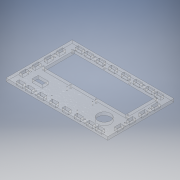
# Autodesk Inventor part: case_top
Saved by Autodesk Inventor 2019 (Build 230136000, 136)
## iProperties
Created: 2019-02-02
Part Number: case_top
Material: Acrylic, Clear
Document SubType Name: Modeling
Designer: suchanek
Density: 1.19 g/cm^3
Appearance: Transparent - Clear
Author: suchanek
Autodesk Inventor part; units mm, degrees
ref_plane "YZ Plane" through (0, 0, 0) normal (1, 0, 0) x (0, 1, 0)
ref_plane "XZ Plane" through (0, 0, 0) normal (0, 1, 0) x (-1, 0, 0)
ref_plane "XY Plane" through (0, 0, 0) normal (0, 0, 1) x (1, 0, 0)
sketch "Sketch1" plane through (0, 0, 0) normal (0, 1, 0) x (-1, 0, 0)
  line L0 (100, 65) -> (-100, 65)
  line L1 (-100, 65) -> (-100, -65)
  line L2 (-100, -65) -> (100, -65)
  line L3 (100, -65) -> (100, 65)
  line L4 (100, 65) -> (-100, -65) construction
  line L5 (-100, 65) -> (100, -65) construction
  line L6 (0, 0) -> (4.5236, 0)
  line L7 (0, 8) -> (0, -20)
  line L8 (0, 0) -> (5.2635, 0)
  line L9 (96, -42) -> (90, -42)
  line L10 (90, -42) -> (90, -30)
  line L11 (90, -30) -> (96, -30)
  line L12 (96, -30) -> (96, -42)
  line L13 (96, -18) -> (90, -18)
  line L14 (90, -18) -> (90, -6)
  line L15 (90, -6) -> (96, -6)
  line L16 (96, -6) -> (96, -18)
  line L17 (66, -55) -> (54, -55)
  line L18 (54, -55) -> (54, -61)
  line L19 (54, -61) -> (66, -61)
  line L20 (66, -61) -> (66, -55)
  line L21 (42, -55) -> (30, -55)
  line L22 (30, -55) -> (30, -61)
  line L23 (30, -61) -> (42, -61)
  line L24 (42, -61) -> (42, -55)
  line L25 (18, -55) -> (6, -55)
  line L26 (6, -55) -> (6, -61)
  line L27 (6, -61) -> (18, -61)
  line L28 (18, -61) -> (18, -55)
  line L29 (72, -61) -> (84, -61)
  line L30 (84, -61) -> (84, -55)
  line L31 (84, -55) -> (72, -55)
  line L32 (72, -55) -> (72, -61)
  line L33 (-96, -42) -> (-90, -42)
  line L34 (-90, -42) -> (-90, -30)
  line L35 (-90, -30) -> (-96, -30)
  line L36 (-96, -30) -> (-96, -42)
  line L37 (-96, -18) -> (-90, -18)
  line L38 (-90, -18) -> (-90, -6)
  line L39 (-90, -6) -> (-96, -6)
  line L40 (-96, -6) -> (-96, -18)
  line L41 (-66, -55) -> (-54, -55)
  line L42 (-54, -55) -> (-54, -61)
  line L43 (-54, -61) -> (-66, -61)
  line L44 (-66, -61) -> (-66, -55)
  line L45 (-42, -55) -> (-30, -55)
  line L46 (-30, -55) -> (-30, -61)
  line L47 (-30, -61) -> (-42, -61)
  line L48 (-42, -61) -> (-42, -55)
  line L49 (-18, -55) -> (-6, -55)
  line L50 (-6, -55) -> (-6, -61)
  line L51 (-6, -61) -> (-18, -61)
  line L52 (-18, -61) -> (-18, -55)
  line L53 (-72, -61) -> (-84, -61)
  line L54 (-84, -61) -> (-84, -55)
  line L55 (-84, -55) -> (-72, -55)
  line L56 (-72, -55) -> (-72, -61)
  line L57 (96, 42) -> (90, 42)
  line L58 (90, 42) -> (90, 30)
  line L59 (90, 30) -> (96, 30)
  line L60 (96, 30) -> (96, 42)
  line L61 (96, 18) -> (90, 18)
  line L62 (90, 18) -> (90, 6)
  line L63 (90, 6) -> (96, 6)
  line L64 (96, 6) -> (96, 18)
  line L65 (66, 55) -> (54, 55)
  line L66 (54, 55) -> (54, 61)
  line L67 (54, 61) -> (66, 61)
  line L68 (66, 61) -> (66, 55)
  line L69 (42, 55) -> (30, 55)
  line L70 (30, 55) -> (30, 61)
  line L71 (30, 61) -> (42, 61)
  line L72 (42, 61) -> (42, 55)
  line L73 (18, 55) -> (6, 55)
  line L74 (6, 55) -> (6, 61)
  line L75 (6, 61) -> (18, 61)
  line L76 (18, 61) -> (18, 55)
  line L77 (72, 61) -> (84, 61)
  line L78 (84, 61) -> (84, 55)
  line L79 (84, 55) -> (72, 55)
  line L80 (72, 55) -> (72, 61)
  line L81 (-90, 30) -> (-96, 30)
  line L82 (-96, 18) -> (-90, 18)
  line L83 (-90, 18) -> (-90, 6)
  line L84 (-90, 6) -> (-96, 6)
  line L85 (-96, 6) -> (-96, 18)
  line L86 (-96, 42) -> (-90, 42)
  line L87 (-96, 30) -> (-96, 42)
  line L88 (-90, 42) -> (-90, 30)
  line L89 (-84, 55) -> (-72, 55)
  line L90 (-84, 61) -> (-84, 55)
  line L91 (-72, 61) -> (-84, 61)
  line L92 (-72, 55) -> (-72, 61)
  line L93 (-66, 61) -> (-66, 55)
  line L94 (-54, 55) -> (-54, 61)
  line L95 (-54, 61) -> (-66, 61)
  line L96 (-66, 55) -> (-54, 55)
  line L97 (-6, 55) -> (-6, 61)
  line L98 (-18, 55) -> (-6, 55)
  line L99 (-6, 61) -> (-18, 61)
  line L100 (-18, 61) -> (-18, 55)
  line L101 (-30, 55) -> (-30, 61)
  line L102 (-42, 61) -> (-42, 55)
  line L103 (-30, 61) -> (-42, 61)
  line L104 (-42, 55) -> (-30, 55)
  line L105 (80, -50) -> (-80, -50)
  line L106 (-80, -50) -> (-80, 10)
  line L107 (-80, 10) -> (80, 10)
  line L108 (80, 10) -> (80, -50)
  circle A0 centre (-63, 35) radius 12.5
  line L109 (73, 41) -> (53, 41)
  line L110 (53, 41) -> (53, 29)
  line L111 (53, 29) -> (73, 29)
  line L112 (73, 29) -> (73, 41)
  line L113 (73, 41) -> (53, 29) construction
  line L114 (53, 41) -> (73, 29) construction
  circle A1 centre (25, 50) radius 0.8
  circle A2 centre (25, 20) radius 0.8
  circle A3 centre (-25, 50) radius 0.8
  circle A4 centre (-25, 20) radius 0.8
  circle A5 centre (83, -48.5) radius 1.5
  circle A6 centre (-25, -53) radius 1.5
  circle A7 centre (-83, -48.5) radius 1.5
  line L115 (0, -20) -> (17.6, -20)
  circle A8 centre (83, 8.5) radius 1.5
  circle A9 centre (-25, 13) radius 1.5
  circle A10 centre (-83, 8.5) radius 1.5
  circle A11 centre (25, -53) radius 1.5
  circle A12 centre (25, 13) radius 1.5
  circle A13 centre (93, 24) radius 1.5
  circle A14 centre (48, 58) radius 1.5
  circle A15 centre (93, -24) radius 1.5
  circle A16 centre (48, -58) radius 1.5
  circle A17 centre (-93, 24) radius 1.5
  circle A18 centre (-48, 58) radius 1.5
  circle A19 centre (-48, -58) radius 1.5
  circle A20 centre (-93, -24) radius 1.5
  point P0 (0, 0)
  point P1 (0, 0)
  point P2 (63, 35)
  point P3 (63, 35)
  dimension "d0" = 130
  dimension "d1" = 200
  dimension "d31" = 6
  dimension "d32" = 4
  dimension "d34" = 6
  dimension "d35" = 12
  dimension "d36" = 12
  dimension "d37" = 12
  dimension "d38" = 6
  dimension "d39" = 12
  dimension "d40" = 12
  dimension "d41" = 12
  dimension "d42" = 12
  dimension "d43" = 12
  dimension "d44" = 6
  dimension "d45" = 12
  dimension "d46" = 6
  dimension "d47" = 4
  dimension "d58" = 160
  dimension "d59" = 60
  dimension "d60" = 15
  dimension "d61" = 20
  dimension "d66" = 25
  dimension "d67" = 20
  dimension "d68" = 27
  dimension "d69" = 20
  dimension "d70" = 12
  dimension "d73" = 27
  dimension "d74" = 50
  dimension "d75" = 5
  dimension "d76" = 10
  dimension "d77" = 1.6
  dimension "d78" = 3
  dimension "d80" = 3
  dimension "d81" = 3
  dimension "d82" = 3
  dimension "d83" = 25
  dimension "d84" = 3
  dimension "d85" = 6
  dimension "d86" = 3
  dimension "d87" = 6
  constraints: 232 end point, 85 symmetric about line, 21 centre point, 21 point on line, 18 parallel, 12 horizontal, 9 midpoint, 9 perpendicular, 5 equal radius, 3 collinear, 2 horizontal alignment, 1 tangent, 1 vertical, 1 vertical alignment, 14 other
  measures "d0" distance of L2.end L0.start
  measures "d1" distance of L1.end L2.end
  measures "d31" distance between parallel lines of L14 L16
  measures "d32" distance between parallel lines of L3 L16
  measures "d34" distance between parallel lines of L15 L8
  measures "d35" distance of L15.end L13.start
  measures "d36" distance between parallel lines of L13 L11
  measures "d37" distance of L11.end L9.start
  measures "d38" distance between parallel lines of L26 L7
  measures "d39" distance of L26.end L27.end
  measures "d40" distance between parallel lines of L28 L22
  measures "d41" distance of L21.start L21.end
  measures "d42" distance between parallel lines of L24 L18
  measures "d43" distance of L17.start L17.end
  measures "d44" distance between parallel lines of L20 L32
  measures "d45" distance of L30.end L31.end
  measures "d46" distance of L25.end L26.end
  measures "d47" distance between parallel lines of L2 L27
  measures "d58" distance of L106.end L107.end
  measures "d59" distance of L105.end L106.end
  measures "d60" distance between parallel lines of L2 L105
  measures "d61" distance between parallel lines of L1 L106
  measures "d66" diameter of A0
  measures "d67" distance from line of L104 A0.centre
  measures "d68" distance from line of L88 A0.centre
  measures "d69" distance of L111.end L110.end
  measures "d70" distance of L110.end L109.end
  measures "d73" distance from line of point (63, 35) L58
  measures "d74" distance of A4.centre A2.centre
  measures "d75" distance from line of L104 A3.centre
  measures "d76" distance from line of L107 A4.centre
  measures "d77" diameter of A1
  measures "d78" diameter of A5
  measures "d80" distance from line of L105 A6.centre
  measures "d81" distance from line of L108 A5.centre
  measures "d82" distance from line of L106 A7.centre
  measures "d83" distance from line of L7 A6.centre
  measures "d84" distance from line of A14.centre L67
  measures "d85" distance from line of A14.centre L66
  measures "d86" distance from line of L58 A13.centre
  measures "d87" distance from line of L59 A13.centre
extrude "Extrusion3" add sketch "Sketch1" along normal blind 6
body "Solid3"
